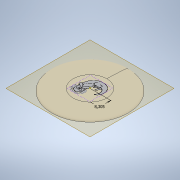
# Autodesk Inventor part: case_top
Saved by Autodesk Inventor 2021 (Build 250183000, 183)
## iProperties
Created: 2021-03-07
Part Number: case_top
Material: Generisch
Document SubType Name: Modeling
Designer: JanHenrik
Density: 1 g/cm^3
Appearance: Vorgabe
Author: JanHenrik
Autodesk Inventor part; units mm, degrees
ref_plane "YZ Plane" through (0, 0, 0) normal (1, 0, 0) x (0, 1, 0)
ref_plane "XY Plane" through (0, 0, 0) normal (0, 0, 1) x (1, 0, 0)
sketch "Skizze1" plane through (0, 0, 0) normal (1, 0, 0) x (0, 1, 0)
  line L0 (0, 0) -> (0, -25)
  line L1 (0, -25) -> (0, -25)
  line L2 (0, -25) -> (0, -25.3)
  line L3 (0, -25.3) -> (0.4, -25.3)
  line L4 (0.4, -25.3) -> (0.4, -27.3)
  line L5 (0, 0) -> (2, 0)
  line L6 (2, 0) -> (2, -12)
  spline S0 degree 4 poles (0.4, -27.3) (1.1095, -26.9423) (1.1714, -26.4773) (1.6189, -23.6497) (1.9462, -13.3271) (2.0016, -12.6963) (2, -12) knots 0 0 0 0 0 0.392472 0.561015 1 1 1 1 1
  line L7 (1.8731, -15.6322) -> (2.0147, -12.051) construction
  arc A0 (1.8861, -15.274) -> (1.9994, -12.409) centre (-927.9256, 22.9329) ccw construction
  line L8 (1.1669, -26.6596) -> (1.4925, -23.5314) construction
  arc A1 (1.1773, -26.3437) -> (1.4376, -23.8427) centre (-33.7592, -21.4436) ccw construction
  point P0 (1.0005, -26.7671)
  point P1 (1.3297, -25.0955)
  point P2 (1.9439, -13.8416)
  dimension "d0" = 25
  dimension "d2" = 0
  dimension "d3" = 0.4
  dimension "d4" = 2
  dimension "d5" = 2
  dimension "d6" = 12
  constraints: 18 end point, 4 midpoint, 4 perpendicular, 2 centre point, 2 horizontal, 2 point on circle, 1 vertical, 9 other
  measures "d0" distance of L0.start L0.end
  measures "d2" distance between parallel lines of L0 L2
  measures "d3" distance between parallel lines of L4 L2
  measures "d4" distance of L3.end L4.end
  measures "d5" distance of L0.start L5.end
  measures "d6" distance of L5.end L6.end
revolve "Umdrehung1" add sketch "Skizze1" angle 360 about axis through (0, 0, 0) along (0, 1, 0)
ref_plane "Arbeitsebene2" through (0, 2, 0) normal (0, 1, 0) x (-1, 0, 0)
sketch "Skizze3" plane through (0, 2, 0) normal (0, 1, 0) x (-1, 0, 0)
  line L0 (-8.1245, 8.305) -> (8.1249, 8.305) construction
  line L1 (8.1249, 8.305) -> (8.1249, -8.3263) construction
  line L2 (8.1249, -8.3263) -> (-8.1245, -8.3263) construction
  line L3 (-8.1245, -8.3263) -> (-8.1245, 8.305) construction
  point P0 (0, 0)
  dimension "d11" = 8.305
  constraints: 2 other
  measures "d11" distance from line of L0 point (0, 0)
